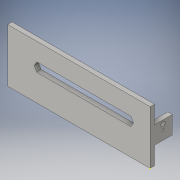
# Autodesk Inventor part: Plate add on
Saved by Autodesk Inventor 2016 (Build 200138000, 138)
## iProperties
Created: 2016-02-22
Part Number: Plate add on
Material: Generic
Document SubType Name: Modeling
Designer: Admin
Density: 1 g/cm^3
Appearance: Default
Author: Admin
Autodesk Inventor part; units mm, degrees
ref_plane "YZ Plane" through (0, 0, 0) normal (1, 0, 0) x (0, 1, 0)
ref_plane "XZ Plane" through (0, 0, 0) normal (0, 1, 0) x (-1, 0, 0)
ref_plane "XY Plane" through (0, 0, 0) normal (0, 0, 1) x (1, 0, 0)
sketch "Sketch1" plane through (0, 0, 0) normal (0, 1, 0) x (-1, 0, 0)
  line L0 (0, 0) -> (0, -6.35)
  line L1 (0, -6.35) -> (203.2, -6.35)
  line L2 (203.2, -6.35) -> (203.2, 0)
  line L3 (203.2, 0) -> (0, 0)
  dimension "d0" = 6.35
  dimension "d1" = 203.2
  constraints: 8 end point, 3 perpendicular, 1 vertical
  measures "d0" distance of L0.start L0.end
  measures "d1" distance of L0.end L1.end
extrude "Extrusion1" add sketch "Sketch1" along normal blind 76.2
sketch "Sketch2" plane through (-203.2, 0, 0) normal (0, 0, 1) x (1, 0, 0)
  line L0 (172.212, 50.8) -> (45.212, 50.8)
  line L1 (45.212, 50.8) -> (45.212, 38.1)
  line L2 (45.212, 38.1) -> (172.212, 38.1)
  line L3 (172.212, 38.1) -> (172.212, 50.8)
  line L4 (45.212, 50.8) -> (-15.6643, 42.2552)
  line L5 (-15.6643, 42.2552) -> (-14.2327, 32.0558)
  line L6 (-14.2327, 32.0558) -> (46.6436, 40.6006)
  line L7 (46.6436, 40.6006) -> (45.212, 50.8)
  line L8 (0, 76.2) -> (203.2, 76.2) projected
  line L9 (203.2, 0) -> (203.2, 76.2) projected
  dimension "d4" = 127
  dimension "d5" = 12.7
  dimension "d24" = 25.4
  dimension "d25" = 30.988
  constraints: 16 end point, 4 parallel, 2 perpendicular, 1 horizontal
  measures "d4" distance of L2.end L1.end
  measures "d5" distance of L1.end L0.end
  measures "d24" distance between parallel lines of L8 L0
  measures "d25" distance between parallel lines of L9 L3
sketch "Sketch3" plane through (-203.2, 0, 0) normal (0, 0, 1) x (1, 0, 0)
  point P0 (203.2, 0)
extrude "Extrusion2" cut sketch "Sketch2" against normal blind 6.35 contours L3 L2 L1 L6 L7 L0 | L7 L6 L1
sketch "Sketch4" plane through (-203.2, 0, 0) normal (0, 0, 1) x (1, 0, 0)
  point P0 (203.2, 0)
sketch "Sketch5" plane through (0, 0, -6.35) normal (0, 0, -1) x (-1, 0, 0)
  line L0 (0, 0) -> (0, 76.2) projected
  line L1 (0, 76.2) -> (6.35, 76.2)
  line L2 (6.35, 76.2) -> (6.35, 25.4)
  line L3 (6.35, 25.4) -> (0, 25.4)
  line L4 (0, 25.4) -> (0, 76.2)
  line L5 (0, 76.2) -> (203.2, 76.2) projected
  line L6 (0, 76.2) -> (6.35, 76.2)
  line L7 (6.35, 76.2) -> (6.35, 50.8)
  line L8 (6.35, 50.8) -> (0, 50.8)
  line L9 (0, 50.8) -> (0, 76.2)
  dimension "d8" = 6.35
  dimension "d9" = 50.8
  dimension "d11" = 25.4
  constraints: 16 end point, 4 parallel, 2 horizontal, 2 perpendicular, 1 midpoint
  measures "d8" distance of L2.end L3.end
  measures "d9" distance of L1.end L2.end
  measures "d11" distance of L6.end L7.end
extrude "Extrusion3" add sketch "Sketch5" along normal blind 25.4 contours L0 L8 L2 L3
sketch "Sketch6" plane through (-6.35, 25.4, -6.35) normal (-1, 0, 0) x (0, 0, 1)
  circle A0 centre (-11.9648, 20.32) radius 3.175
  circle A1 centre (-11.9648, 12.7) radius 1.5875
  line L0 (0, 0) -> (-25.4, 0) projected
  line L1 (-25.4, 25.4) -> (0, 25.4) projected
  point P0 (6.35, -25.4)
  dimension "d14" = 6.35
  dimension "d15" = 3.175
  dimension "d16" = 12.7
  dimension "d17" = 5.08
  constraints: 2 centre point
  measures "d14" diameter of A0
  measures "d15" diameter of A1
  measures "d16" distance from line of L0 A1.centre
  measures "d17" distance from line of L1 A0.centre
extrude "Extrusion4" cut sketch "Sketch6" against normal blind 6.35
sketch "Sketch7" plane through (0, 0, -6.35) normal (0, 0, -1) x (-1, 0, 0)
  line L0 (30.988, 38.1) -> (30.988, 50.8) projected
  line L1 (23.6557, 44.45) -> (27.3218, 50.8)
  line L2 (27.3218, 50.8) -> (34.6542, 50.8)
  line L3 (34.6542, 50.8) -> (38.3203, 44.45)
  line L4 (38.3203, 44.45) -> (34.6542, 38.1)
  line L5 (34.6542, 38.1) -> (27.3218, 38.1)
  line L6 (27.3218, 38.1) -> (23.6557, 44.45)
  line L7 (157.988, 50.8) -> (157.988, 38.1) projected
  line L8 (150.6557, 44.45) -> (154.3218, 50.8)
  line L9 (154.3218, 50.8) -> (161.6542, 50.8)
  line L10 (161.6542, 50.8) -> (165.3203, 44.45)
  line L11 (165.3203, 44.45) -> (161.6542, 38.1)
  line L12 (161.6542, 38.1) -> (154.3218, 38.1)
  line L13 (154.3218, 38.1) -> (150.6557, 44.45)
  point P0 (0, 0)
  point P1 (30.988, 44.45)
  point P2 (157.988, 44.45)
  dimension "d20" = 12.7
  dimension "d21" = 12.7
  constraints: 24 end point, 2 midpoint, 26 other
  measures "d20" distance between parallel lines of L5 L2
  measures "d21" distance between parallel lines of L12 L9
extrude "Extrusion5" cut sketch "Sketch7" against normal blind 6.35
body "Solid1"
